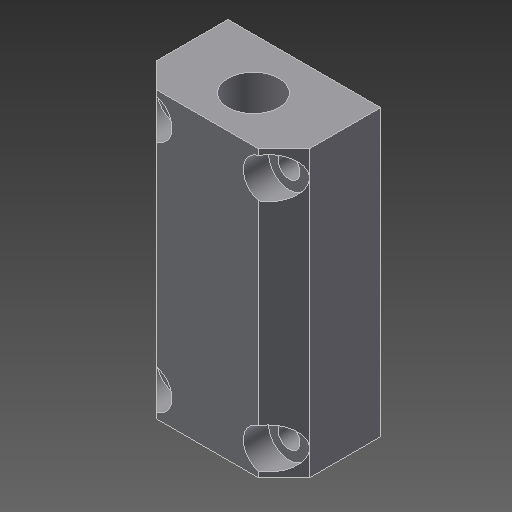
# Autodesk Inventor part: MHCAW10
Saved by Autodesk Inventor 2021.1 (Build 251245010, 245A)
## iProperties
Created: 2008-11-14
Part Number: MHCAW10
Material: MISUMI
Document SubType Name: Modeling
Density: 1 g/cm^3
Mass: 24.5904 g
Surface Area: 87.581 cm^2
Volume: 24.5904 cm^3
Appearance: 既定
Title: 無給油ブシュハウジングユニット
Autodesk Inventor part; units mm, degrees
ref_plane "YZ Plane" through (0, 0, 0) normal (1, 0, 0) x (0, 1, 0)
ref_plane "XZ Plane" through (0, 0, 0) normal (0, 1, 0) x (-1, 0, 0)
ref_plane "XY Plane" through (0, 0, 0) normal (0, 0, 1) x (1, 0, 0)
sketch "スケッチ1" plane through (0, 0, 0) normal (0, 0, 1) x (1, 0, 0)
  line L0 (-15, 28) -> (15, 28)
  line L1 (15, 28) -> (15, -28)
  line L2 (15, -28) -> (-15, -28)
  line L3 (-15, -28) -> (-15, 28)
  point P0 (0, 0)
  point P1 (15, 0)
  point P2 (0, -28)
  dimension "d0" = 30
  dimension "d1" = 56
  constraints: 8 end point, 2 midpoint, 2 parallel, 1 horizontal, 1 horizontal alignment, 1 perpendicular, 1 vertical alignment
  measures "d0" distance of L1.end L2.end
  measures "d1" distance of L2.end L0.start
extrude "押し出し1" add sketch "スケッチ1" along normal blind 19
sketch "スケッチ2" plane through (0, 0, 19) normal (0, 0, 1) x (1, 0, 0)
  line L0 (-15, -28) -> (-15, 28) projected
  line L1 (15, -28) -> (-15, -28) projected
  point P0 (0, 0)
  point P1 (-11, -23)
  dimension "d4" = 4
  dimension "d5" = 5
  measures "d4" distance from line of point (-11, -23) L0
  measures "d5" distance from line of point (-11, -23) L1
hole "穴1" at (-11, -23, 19) direction (0, 0, -1) diameter 4.3 end through all counterbore diameter 8 counterbore depth 5
pattern_linear "矩形状パターン1" count 2 spacing 22 along (1, 0, 0) count 2 spacing 46 along (0, 1, 0) of "穴1"
sketch "スケッチ3" plane through (-15, 28, 0) normal (0, 1, 0) x (1, 0, 0)
  line L0 (0, 0) -> (30, 0) projected
  point P0 (15, 0)
  point P1 (15, -10)
  point P2 (15, 0)
  dimension "d19" = 10
  constraints: 1 midpoint, 1 vertical alignment
  measures "d19" distance from line of point (15, -10) L0
hole "穴2" at (0, 28, 10) direction (0, -1, 0) diameter 10 end through all
sketch "スケッチ4" plane through (-15, 28, 0) normal (0, 1, 0) x (1, 0, 0)
  line L0 (0, -19) -> (30, -19) projected
  line L1 (0, 0) -> (0, -19) projected
  line L2 (0, -14) -> (5, -19)
  point P0 (15, 0)
  dimension "d30" = 5
  dimension "d31" = 5
  constraints: 2 end point, 2 point on line
  measures "d30" distance from line of L2.end L1
  measures "d31" distance from line of L2.start L0
extrude "押し出し2" cut sketch "スケッチ4" against normal through all
mirror "ミラー1" about plane through (0, 0, 0) normal (1, 0, 0) of "押し出し2"
